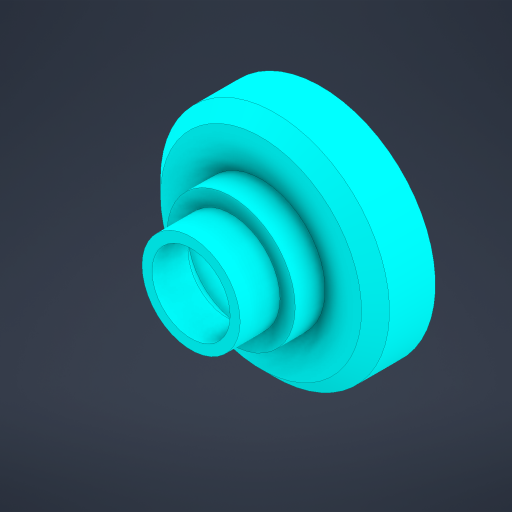
# Autodesk Inventor part: Filter Adapter (SM1)
Saved by Autodesk Inventor 2023.4 (Build 274418000, 418)
## iProperties
Created: 2024-05-15
Part Number: Filter Adapter (SM1)
Material: Generic
Document SubType Name: Modeling
Designer: xSibe
Density: 1 g/cm^3
Appearance: Plastic Cyan
Author: xSibe
Autodesk Inventor part; units mm, degrees
ref_plane "YZ Plane" through (0, 0, 0) normal (1, 0, 0) x (0, 1, 0)
ref_plane "XZ Plane" through (0, 0, 0) normal (0, 1, 0) x (-1, 0, 0)
ref_plane "XY Plane" through (0, 0, 0) normal (0, 0, 1) x (1, 0, 0)
sketch "Sketch1" plane through (0, 0, 0) normal (0, 0, 1) x (1, 0, 0)
  circle A0 centre (0, 0) radius 6.1437
  circle A1 centre (0, 0) radius 4.8937
  circle A2 centre (0, 0) radius 13.0938
  circle A3 centre (0, 0) radius 6.7838
  circle A4 centre (0, 0) radius 14.3438
  circle A5 centre (0, 0) radius 8.0337
  dimension "d0" = 12.2875
  dimension "d1" = 1.25
  dimension "d4" = 26.1875
  dimension "d5" = 13.5675
  dimension "d6" = 1.25
  dimension "d7" = 1.25
  constraints: 6 centre point, 3 coincident
  measures "d0" diameter of A0
  measures "d1" radial gap between concentric circles of A0 A1
  measures "d4" diameter of A2
  measures "d5" diameter of A3
  measures "d6" radial gap between concentric circles of A2 A4
  measures "d7" radial gap between concentric circles of A3 A5
extrude "Extrusion1" add sketch "Sketch1" along normal blind 5 contours A0
extrude "Extrusion2" add sketch "Sketch1" against normal blind 1.25 contours A0 | A3 | A5
extrude "Extrusion3" add sketch "Sketch1" against normal blind 2.5 from surface at -1.25 contours A5
extrude "Extrusion4" add sketch "Sketch1" against normal blind 2.5 from surface at -3.75 contours A2 | A4 | A5
extrude "Extrusion5" add sketch "Sketch1" against normal blind 5 from surface at -6.25 contours A4
chamfer "Chamfer1" distance 1.75 angle 45 3 edges at (-4.8937, 0, -1.25) (-6.7838, 0, -6.25) (-14.3438, 0, -3.75)
body "Solid1"
